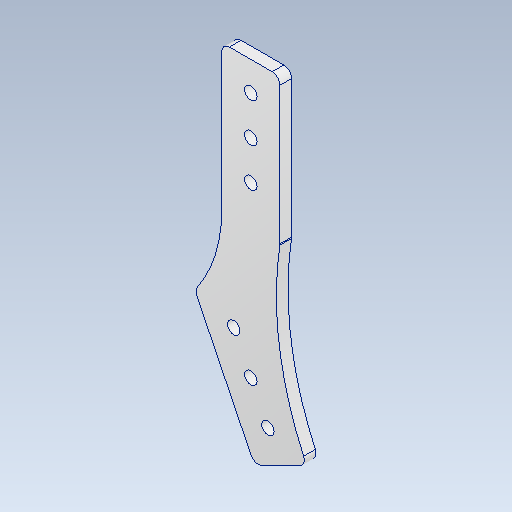
# Autodesk Inventor part: オムニ_固定具寸法不明2
Saved by Autodesk Inventor 2021 (Build 250183000, 183)
## iProperties
Created: 2022-02-03
Part Number: オムニ_固定具寸法不明2
Material: アルミニウム 6061
Document SubType Name: Modeling
Designer: hirohumi
Density: 2.7 g/cm^3
Appearance: アルミニウム - フラット
Mass: 11.0913 g
Surface Area: 35.3748 cm^2
Volume: 4.10789 cm^3
Author: hirohumi
Autodesk Inventor part; units mm, degrees
ref_plane "YZ Plane" through (0, 0, 0) normal (1, 0, 0) x (0, 1, 0)
ref_plane "XZ Plane" through (0, 0, 0) normal (0, 1, 0) x (-1, 0, 0)
ref_plane "XY Plane" through (0, 0, 0) normal (0, 0, 1) x (1, 0, 0)
sketch "スケッチ1" plane through (0, 0, 0) normal (0, 0, 1) x (1, 0, 0)
  circle A0 centre (11.8968, -42.422) radius 1.6 projected
  circle A1 centre (7.5, -33.4405) radius 1.6 projected
  circle A2 centre (3.1032, -24.4589) radius 1.6 projected
  circle A3 centre (7.5, 10) radius 1.6 projected
  circle A4 centre (7.5, 20) radius 1.6 projected
  circle A5 centre (7.5, 30) radius 1.6 projected
  line L0 (-6.9305, -21.0203) -> (8.4582, -52.4558)
  line L1 (8.4582, -52.4558) -> (21.9305, -45.8606)
  line L2 (15, 0) -> (15, 37.5)
  line L3 (15, 37.5) -> (0, 37.5)
  line L4 (0, 37.5) -> (0, 0)
  arc A6 (15, 0) -> (21.9305, -45.8606) centre (91.2366, -11.933) ccw
  line L5 (21.9305, -45.8606) -> (6.5418, -14.4252) construction
  arc A7 (-6.9305, -21.0203) -> (0, 0) centre (-35.3427, 0) ccw
  line L6 (6.5418, -14.4252) -> (-6.9305, -21.0203) construction
  dimension "d0" = 7.5
  dimension "d1" = 7.5
  dimension "d2" = 7.5
  dimension "d3" = 7.5
  dimension "d4" = 7.5
  dimension "d5" = 7.5
  dimension "d6" = 7.5
  constraints: 14 end point, 4 point on circle, 3 perpendicular, 2 centre point, 2 tangent, 2 vertical, 1 horizontal alignment, 1 parallel
  measures "d0" distance from line of L3 A5.centre
  measures "d1" distance from line of A5.centre L2
  measures "d2" distance from line of L0 A0.centre
  measures "d3" distance from line of L0 A2.centre
  measures "d4" distance from line of A0.centre L1
  measures "d5" distance from line of A1.centre L5
  measures "d6" distance from line of A2.centre L6
extrude "押し出し1" add sketch "スケッチ1" along normal blind 3
fillet "フィレット1" radius 2 6 edges at (21.9305, -45.8606, 1.5) (8.4582, -52.4558, 1.5) (-6.9305, -21.0203, 1.5) (0, 37.5, 1.5) (15, 37.5, 1.5) (15, 0, 1.5)
